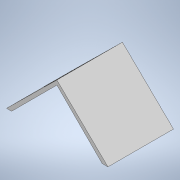
# Autodesk Inventor part: TABLERO
Saved by Autodesk Inventor 2022 (Build 260153000, 153)
## iProperties
Created: 2022-08-26
Part Number: TABLERO
Material: Genérico
Document SubType Name: Modeling
Designer: Usuario
Density: 1 g/cm^3
Appearance: Valor por defecto
Author: Usuario
Autodesk Inventor part; units mm, degrees
ref_plane "YZ Plane" through (0, 0, 0) normal (1, 0, 0) x (0, 1, 0)
ref_plane "XZ Plane" through (0, 0, 0) normal (0, 1, 0) x (-1, 0, 0)
sketch "Boceto2" plane through (0, 0, 0) normal (0, 0, 1) x (1, 0, 0)
  line L0 (0, 0) -> (196, 0)
  line L1 (0, 0) -> (-196, 0)
  line L2 (0, 0) -> (0, 215)
  line L3 (-196, 0) -> (-218, 0)
  line L4 (-218, 0) -> (0, 215)
  line L5 (-263.5923, -44.9649) -> (-252.2786, -56.2786)
  line L6 (-263.5923, -44.9649) -> (-247.5923, -44.9649) construction
  line L7 (-252.2786, -56.2786) -> (0, 196)
  line L8 (-252.2786, -56.2786) -> (-196, 0)
  line L9 (196, 0) -> (221, 0)
  line L10 (221, 0) -> (0, 215)
  line L11 (117.9791, 100.2239) -> (106.6654, 88.9102)
  line L12 (117.9791, 100.2239) -> (133.9791, 100.2239) construction
  line L13 (106.6654, 88.9102) -> (0, 196)
  line L14 (106.6654, 88.9102) -> (196, 0)
  dimension "d0" = 196
  dimension "d1" = 196
  dimension "d2" = 215
  dimension "d3" = 22
  dimension "d4" = 16
  dimension "d5" = 45
  dimension "d6" = 25
  dimension "d7" = 16
  dimension "d8" = 135
  constraints: 30 end point, 6 horizontal, 3 point on line, 2 equal length, 1 collinear, 1 perpendicular, 1 vertical
  measures "d0" distance of L0.start L0.end
  measures "d1" distance of L0.start L1.end
  measures "d2" distance of L0.start L2.end
  measures "d3" distance of L1.end L3.end
  measures "d4" distance of L5.start L5.end
  measures "d5" angle of L5 L6
  measures "d6" distance of L0.end L9.end
  measures "d7" distance of L11.start L11.end
  measures "d8" angle of L11 L12
extrude "Extrusión1" add sketch "Boceto2" against normal blind 283.5 contours L14 L11 L10 L9 | L3 L4 L2 L7 | L2 L10 L11 L13
ref_plane "Plano de trabajo1" through (0, 215, -283.5) normal (0.7021908, -0.7119888, 0) x (0, 0, 1)
sketch "Boceto3" plane through (0, 215, -283.5) normal (0.7021908, -0.7119888, 0) x (0, 0, 1)
  line L0 (283.5, 150.971) -> (0, 150.971)
  line L1 (0, 306.1846) -> (0, 0) projected
  line L2 (283.5, -6.3785) -> (0, -6.3785) projected
  line L3 (141.75, 150.971) -> (141.75, 0)
  line L4 (283.5, 0) -> (0, 0) projected
  line L5 (141.75, 0) -> (141.75, 80)
  line L6 (121.75, 80) -> (51.75, 80)
  line L7 (51.75, 80) -> (51.75, 220)
  line L8 (51.75, 220) -> (121.75, 220)
  line L9 (121.75, 200) -> (71.75, 200)
  line L10 (71.75, 200) -> (71.75, 100)
  line L11 (71.75, 100) -> (121.75, 100)
  line L12 (141.75, 80) -> (161.75, 80)
  line L13 (181.75, 220) -> (141.75, 100)
  line L14 (221.75, 80) -> (181.75, 220)
  line L15 (221.75, 80) -> (201.75, 80)
  line L16 (201.75, 80) -> (181.75, 150.971)
  line L17 (161.75, 80) -> (181.75, 150.971)
  line L18 (141.75, 80) -> (135.0833, 80)
  line L19 (121.75, 80) -> (121.75, 220)
  line L20 (135.0833, 80) -> (142.2633, 101.5399)
  point P0 (141.75, 220)
  point P1 (141.75, 200)
  dimension "d28" = 90
  dimension "d29" = 100
  dimension "d30" = 70
  dimension "d31" = 20
  constraints: 36 end point, 11 point on line, 6 perpendicular, 2 midpoint, 1 horizontal, 1 parallel
  measures "d28" distance of L5.end L6.end
  measures "d29" distance of L9.end L10.end
  measures "d30" distance of L10.end L13.end
  measures "d31" distance of L6.start L5.end
extrude "Extrusión2" cut sketch "Boceto3" along normal blind 1 contours L10 L11 L19 L6 L7 L0 | L0 L7 L8 L19 L9 L10
extrude "Extrusión3" add sketch "Boceto3" against normal blind 1 contours L14 L15 L16 L0 | L0 L13 L14 | L17 L12 L3 L13 L0
